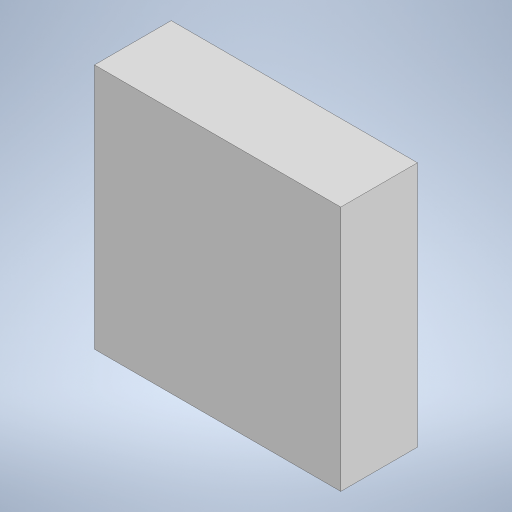
# Autodesk Inventor part: Part_6_lid
Saved by Autodesk Inventor 2023 (Build 270158000, 158)
## iProperties
Created: 2023-10-25
Part Number: Part_6_lid
Material: Generic
Document SubType Name: Modeling
Designer: zskus
Density: 1 g/cm^3
Appearance: Default
Author: zskus
Autodesk Inventor part; units mm, degrees
ref_plane "YZ Plane" through (0, 0, 0) normal (1, 0, 0) x (0, 1, 0)
ref_plane "XZ Plane" through (0, 0, 0) normal (0, 1, 0) x (-1, 0, 0)
ref_plane "XY Plane" through (0, 0, 0) normal (0, 0, 1) x (1, 0, 0)
sketch "Sketch1" plane through (0, 0, 0) normal (0, 0, 1) x (1, 0, 0)
  line L0 (-38.227, 38.227) -> (38.227, 38.227)
  line L1 (38.227, 38.227) -> (38.227, -38.227)
  line L2 (38.227, -38.227) -> (-38.227, -38.227)
  line L3 (-38.227, -38.227) -> (-38.227, 38.227)
  point P0 (0, 0)
  dimension "d0" = 76.454
  dimension "d1" = 76.454
  dimension "d2" = 38.227
  dimension "d3" = 38.227
  constraints: 8 end point, 2 parallel, 1 horizontal, 1 perpendicular
  measures "d0" distance of L0.end L1.end
  measures "d1" distance of L0.start L0.end
  measures "d2" distance from line of point (0, 0) L1
  measures "d3" distance from line of L0 point (0, 0)
extrude "Extrusion1" add sketch "Sketch1" along normal blind 2.54
sketch "Sketch2" plane through (0, 0, 2.54) normal (0, 0, 1) x (1, 0, 0)
  line L0 (-38.227, -38.227) -> (38.227, -38.227) projected
  line L1 (38.227, -38.227) -> (38.227, 38.227) projected
  line L2 (38.227, 38.227) -> (-38.227, 38.227) projected
  line L3 (-38.227, 38.227) -> (-38.227, -38.227) projected
  line L4 (-40.767, 40.767) -> (40.767, 40.767)
  line L5 (40.767, 40.767) -> (40.767, -40.767)
  line L6 (40.767, -40.767) -> (-40.767, -40.767)
  line L7 (-40.767, -40.767) -> (-40.767, 40.767)
  point P0 (0, 0)
  dimension "d6" = 2.54
  constraints: 8 end point, 3 other
  measures "d6" distance between parallel lines of L2 L4
extrude "Extrusion2" add sketch "Sketch2" against normal blind 25.4
equation "\"d2\" = 0.5 * d1"
equation "\"d3\" = 0.5 * d0"
body "Solid1"
